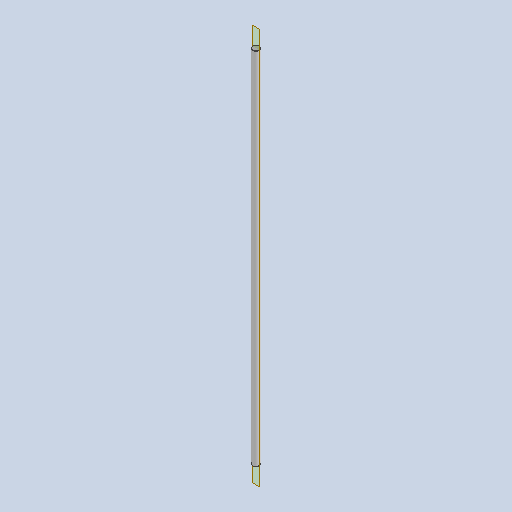
# Autodesk Inventor part: TS_Magazin_Fuehrungselement_int
Saved by Autodesk Inventor 2025.2 (Build 292293000, 293)
## iProperties
Created: 2025-06-01
Part Number: TS_Magazin_Fuehrungselement_int
Material: Generisch
Document SubType Name: Modeling
Designer: tino
Density: 1 g/cm^3
Appearance: Vorgabe
Author: tino
Autodesk Inventor part; units mm, degrees
ref_plane "YZ Plane" through (0, 0, 0) normal (1, 0, 0) x (0, 1, 0)
ref_plane "XY Plane" through (0, 0, 0) normal (0, 0, 1) x (1, 0, 0)
sketch "Skizze2" plane through (0, 0, 0) normal (0, 0, 1) x (1, 0, 0)
  circle A0 centre (0, 0) radius 5
  dimension "d0" = 10
  constraints: 1 centre point, 1 coincident
  measures "d0" diameter of A0
extrude "Extrusion1" add sketch "Skizze2" along normal mid plane 505
sketch "Skizze3" plane through (0, 0, -252.5) normal (0, 0, -1) x (-1, 0, 0)
  point P0 (0, 0)
  point P1 (0, 0)
  constraints: 1 coincident
hole "Bohrung1" at (0, 0, -252.5) direction (0, 0, 1) diameter 4.917 depth 12 tip angle 118 thread size "M6x1" class "6H" standard "ISO Metric profile"
chamfer "Fasen1" distance 0.5 angle 45 3 edges at (0, -2.4585, -252.5) (-5, 0, -252.5) (-5, 0, 252.5)
equation "\"d0\" = Durchmesser_fuehrungsstab"
equation "\"d1\" = Hoehe_Magazin + Fuehrung_Bodenplatte"
equation "\"d4\" = Tiefe_Bohrung"
equation "\"d10\" = Fase"
equation "\"Durchmesser_fuehrungsstab\" = 10"
equation "\"Hoehe_Magazin\" = 500"
equation "\"Tiefe_Bohrung\" = 10"
equation "\"Fuehrung_Bodenplatte\" = 5"
equation "\"Fase\" = 0.5"
